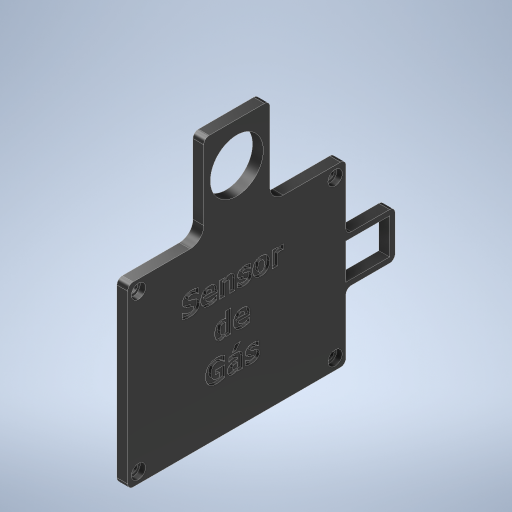
# Autodesk Inventor part: Suporte UNO-tampa
Saved by Autodesk Inventor 2023 (Build 270158000, 158)
## iProperties
Created: 2023-06-01
Part Number: Suporte UNO-tampa
Material: Genérico
Document SubType Name: Modeling
Designer: Inteli
Density: 1 g/cm^3
Appearance: Brilhosa - Preta
Author: Inteli
Autodesk Inventor part; units mm, degrees
ref_plane "YZ Plane" through (0, 0, 0) normal (1, 0, 0) x (0, 1, 0)
ref_plane "XZ Plane" through (0, 0, 0) normal (0, 1, 0) x (-1, 0, 0)
ref_plane "XY Plane" through (0, 0, 0) normal (0, 0, 1) x (1, 0, 0)
sketch "Esboço1" plane through (0, 0, 0) normal (1, 0, 0) x (0, 1, 0)
  line L0 (0, -2) -> (0, -78.8)
  line L1 (2, -80.8) -> (63.8, -80.8)
  line L2 (65.8, -78.8) -> (65.8, -52.65)
  line L3 (2, 0) -> (63.8, 0)
  line L4 (65.8, -2) -> (65.8, -28.15)
  line L5 (65.8, -28.15) -> (96.7, -28.15)
  line L6 (65.8, -52.65) -> (96.7, -52.65)
  line L7 (98.7, -50.65) -> (98.7, -30.15)
  arc A0 (98.7, -30.15) -> (96.7, -28.15) centre (96.7, -30.15) ccw
  arc A1 (96.7, -52.65) -> (98.7, -50.65) centre (96.7, -50.65) ccw
  arc A2 (65.8, -2) -> (63.8, 0) centre (63.8, -2) ccw
  arc A3 (63.8, -80.8) -> (65.8, -78.8) centre (63.8, -78.8) ccw
  arc A4 (0, -78.8) -> (2, -80.8) centre (2, -78.8) ccw
  arc A5 (2, 0) -> (0, -2) centre (2, -2) ccw
  point P0 (0, 0)
  point P1 (0, -80.8)
  point P2 (65.8, -80.8)
  point P3 (65.8, 0)
  point P4 (98.7, -28.15)
  point P5 (98.7, -52.65)
  dimension "d0" = 80.8
  dimension "d1" = 65.8
  dimension "d2" = 28.15
  dimension "d3" = 65.8
  dimension "d4" = 28.15
  dimension "d5" = 32.9
  dimension "d6" = 32.9
  dimension "d7" = 2
  constraints: 16 end point, 12 point on circle, 12 point on line, 12 tangent, 6 centre point, 5 equal radius, 4 horizontal, 2 vertical, 1 perpendicular
  measures "d0" distance of point (0, 0) point (0, -80.8)
  measures "d1" distance of point (0, -80.8) point (65.8, -80.8)
  measures "d2" distance of point (65.8, -80.8) L2.end
  measures "d3" distance of point (0, 0) point (65.8, 0)
  measures "d4" distance of point (65.8, 0) L4.end
  measures "d5" distance of L4.end point (98.7, -28.15)
  measures "d6" distance of L2.end point (98.7, -52.65)
  measures "d7" radius of A0
extrude "Extrusão1" add sketch "Esboço1" along normal blind 4
sketch "Esboço2" plane through (4, 0, 0) normal (1, 0, 0) x (0, 0, -1)
  circle A0 centre (4, 61.8) radius 1.6
  circle A1 centre (76.8, 61.8) radius 1.6
  circle A2 centre (76.8, 4) radius 1.6
  circle A3 centre (4, 4) radius 1.6
  line L0 (0, 63.8) -> (0, 2) projected
  line L1 (28.15, 65.8) -> (2, 65.8) projected
  line L2 (78.8, 65.8) -> (52.65, 65.8) projected
  line L3 (80.8, 2) -> (80.8, 63.8) projected
  line L4 (2, 0) -> (78.8, 0) projected
  circle A4 centre (40.4, 83.9) radius 9.8
  line L5 (50.65, 98.7) -> (30.15, 98.7) projected
  line L6 (52.65, 65.8) -> (52.65, 96.7) projected
  line L7 (28.15, 96.7) -> (28.15, 65.8) projected
  point P0 (0, 0)
  dimension "d10" = 3.2
  dimension "d11" = 3.2
  dimension "d12" = 3.2
  dimension "d13" = 3.2
  dimension "d14" = 4
  dimension "d15" = 4
  dimension "d16" = 4
  dimension "d17" = 4
  dimension "d18" = 4
  dimension "d19" = 4
  dimension "d20" = 4
  dimension "d21" = 4
  dimension "d22" = 19.6
  dimension "d23" = 14.8
  dimension "d24" = 24.5
  dimension "d25" = 12.25
  constraints: 5 centre point
  measures "d10" diameter of A0
  measures "d11" diameter of A1
  measures "d12" diameter of A2
  measures "d13" diameter of A3
  measures "d14" distance from line of L0 A0.centre
  measures "d15" distance from line of L1 A0.centre
  measures "d16" distance from line of L2 A1.centre
  measures "d17" distance from line of L3 A1.centre
  measures "d18" distance from line of L4 A2.centre
  measures "d19" distance from line of L3 A2.centre
  measures "d20" distance from line of L0 A3.centre
  measures "d21" distance from line of L4 A3.centre
  measures "d22" diameter of A4
  measures "d23" distance from line of L5 A4.centre
  measures "d24" distance between parallel lines of L6 L7
  measures "d25" distance from line of L6 A4.centre
extrude "Extrusão2" cut sketch "Esboço2" against normal through all
sketch "Esboço3" plane through (4, 0, 0) normal (1, 0, 0) x (0, 0, -1)
  circle A0 centre (4, 61.8) radius 1.6 projected
  circle A1 centre (4, 61.8) radius 2.6
  circle A2 centre (76.8, 61.8) radius 1.6 projected
  circle A3 centre (76.8, 61.8) radius 2.65
  circle A4 centre (76.8, 4) radius 1.6 projected
  circle A5 centre (76.8, 4) radius 2.6
  circle A6 centre (4, 4) radius 1.6 projected
  circle A7 centre (4, 4) radius 2.6
  point P0 (0, 0)
  dimension "d28" = 5.2
  dimension "d29" = 5.3
  dimension "d30" = 5.2
  dimension "d31" = 5.2
  constraints: 4 centre point, 4 coincident
  measures "d28" diameter of A1
  measures "d29" diameter of A3
  measures "d30" diameter of A5
  measures "d31" diameter of A7
extrude "Extrusão3" cut sketch "Esboço3" against normal blind 2
sketch "Esboço4" plane through (4, 0, 0) normal (1, 0, 0) x (0, 0, -1)
  line L0 (17.1867, 52.3222) -> (60.1959, 52.3222) construction
  line L1 (60.1959, 52.3222) -> (60.1959, 16.2554) construction
  line L2 (60.1959, 16.2554) -> (17.1867, 16.2554) construction
  line L3 (17.1867, 16.2554) -> (17.1867, 52.3222) construction
  spline S0 degree 2 poles (23.1095, 44.0369) (22.1889, 44.0369) (20.8015, 44.3935) (20.2051, 44.6528) knots 0 0 0 1 2 2 2
  line L4 (20.2051, 44.6528) -> (20.2051, 46.5588)
  line L5 (20.2051, 46.5588) -> (20.3866, 46.5588)
  spline S1 degree 2 poles (20.3866, 46.5588) (20.9896, 46.0467) (22.4353, 45.4956) (23.116, 45.4956) knots 0 0 0 1 2 2 2
  spline S2 degree 2 poles (23.116, 45.4956) (23.291, 45.4956) (23.855, 45.5734) (24.0236, 45.6512) knots 0 0 0 1 2 2 2
  spline S3 degree 2 poles (24.0236, 45.6512) (24.231, 45.742) (24.5228, 46.0726) (24.5228, 46.3384) knots 0 0 0 1 2 2 2
  spline S4 degree 2 poles (24.5228, 46.3384) (24.5228, 46.6431) (24.0495, 47.0191) (23.7254, 47.1034) knots 0 0 0 1 2 2 2
  spline S5 degree 2 poles (23.7254, 47.1034) (23.3169, 47.2136) (22.3899, 47.4016) (21.9814, 47.5442) knots 0 0 0 1 2 2 2
  spline S6 degree 2 poles (21.9814, 47.5442) (21.0544, 47.8684) (20.2505, 48.977) (20.2505, 49.8068) knots 0 0 0 1 2 2 2
  spline S7 degree 2 poles (20.2505, 49.8068) (20.2505, 50.9284) (22.15, 52.3222) (23.5763, 52.3222) knots 0 0 0 1 2 2 2
  spline S8 degree 2 poles (23.5763, 52.3222) (24.2894, 52.3222) (25.7027, 52.0305) (26.2602, 51.7841) knots 0 0 0 1 2 2 2
  line L6 (26.2602, 51.7841) -> (26.2602, 49.9559)
  line L7 (26.2602, 49.9559) -> (26.0852, 49.9559)
  spline S9 degree 2 poles (26.0852, 49.9559) (25.6379, 50.3384) (24.3542, 50.8635) (23.68, 50.8635) knots 0 0 0 1 2 2 2
  spline S10 degree 2 poles (23.68, 50.8635) (23.4142, 50.8635) (22.9993, 50.7857) (22.7659, 50.682) knots 0 0 0 1 2 2 2
  spline S11 degree 2 poles (22.7659, 50.682) (22.5779, 50.5977) (22.3056, 50.2606) (22.3056, 50.0532) knots 0 0 0 1 2 2 2
  spline S12 degree 2 poles (22.3056, 50.0532) (22.3056, 49.742) (22.74, 49.3854) (23.3623, 49.2428) knots 0 0 0 1 2 2 2
  spline S13 degree 2 poles (23.3623, 49.2428) (23.7643, 49.152) (24.5098, 48.977) (24.9377, 48.8279) knots 0 0 0 1 2 2 2
  spline S14 degree 2 poles (24.9377, 48.8279) (25.7675, 48.5232) (26.5779, 47.5118) (26.5779, 46.682) knots 0 0 0 1 2 2 2
  spline S15 degree 2 poles (26.5779, 46.682) (26.5779, 45.4891) (24.7043, 44.0369) (23.1095, 44.0369) knots 0 0 0 1 2 2 2
  spline S16 degree 2 poles (30.5908, 44.0175) (28.8793, 44.0175) (27.0576, 45.6512) (27.0576, 47.1617) knots 0 0 0 1 2 2 2
  spline S17 degree 2 poles (27.0576, 47.1617) (27.0576, 48.6399) (28.7562, 50.4032) (30.2861, 50.4032) knots 0 0 0 1 2 2 2
  spline S18 degree 2 poles (30.2861, 50.4032) (31.667, 50.4032) (33.0673, 48.9057) (33.0673, 47.5183) knots 0 0 0 1 2 2 2
  line L8 (33.0673, 47.5183) -> (33.0673, 46.8376)
  line L9 (33.0673, 46.8376) -> (28.9377, 46.8376)
  spline S19 degree 2 poles (28.9377, 46.8376) (28.9636, 46.4162) (29.2683, 45.8587) (29.5147, 45.6901) knots 0 0 0 1 2 2 2
  spline S20 degree 2 poles (29.5147, 45.6901) (29.7545, 45.5216) (30.4028, 45.3789) (30.7853, 45.3789) knots 0 0 0 1 2 2 2
  spline S21 degree 2 poles (30.7853, 45.3789) (31.1095, 45.3789) (31.7448, 45.5216) (32.0106, 45.6447) knots 0 0 0 1 2 2 2
  spline S22 degree 2 poles (32.0106, 45.6447) (32.244, 45.742) (32.633, 45.9818) (32.7562, 46.0726) knots 0 0 0 1 2 2 2
  line L10 (32.7562, 46.0726) -> (32.9571, 46.0726)
  line L11 (32.9571, 46.0726) -> (32.9571, 44.5167)
  spline S23 degree 2 poles (32.9571, 44.5167) (32.7238, 44.4259) (32.3477, 44.2703) (32.0106, 44.1925) knots 0 0 0 1 2 2 2
  spline S24 degree 2 poles (32.0106, 44.1925) (31.7059, 44.1083) (31.0576, 44.0175) (30.5908, 44.0175) knots 0 0 0 1 2 2 2
  spline S25 degree 2 poles (31.2132, 47.9721) (31.2003, 48.5686) (30.6751, 49.1974) (30.137, 49.1974) knots 0 0 0 1 2 2 2
  spline S26 degree 2 poles (30.137, 49.1974) (29.586, 49.1974) (28.9636, 48.5361) (28.9312, 47.9721) knots 0 0 0 1 2 2 2
  line L12 (28.9312, 47.9721) -> (31.2132, 47.9721)
  line L13 (39.68, 44.1796) -> (37.787, 44.1796)
  line L14 (37.787, 44.1796) -> (37.787, 47.1682)
  spline S27 degree 2 poles (37.787, 47.1682) (37.787, 47.5378) (37.7286, 48.2639) (37.6508, 48.4324) knots 0 0 0 1 2 2 2
  spline S28 degree 2 poles (37.6508, 48.4324) (37.5536, 48.6399) (37.1905, 48.8149) (36.8793, 48.8149) knots 0 0 0 1 2 2 2
  spline S29 degree 2 poles (36.8793, 48.8149) (36.6524, 48.8149) (36.1792, 48.6399) (35.9134, 48.4519) knots 0 0 0 1 2 2 2
  line L15 (35.9134, 48.4519) -> (35.9134, 44.1796)
  line L16 (35.9134, 44.1796) -> (34.0333, 44.1796)
  line L17 (34.0333, 44.1796) -> (34.0333, 50.2152)
  line L18 (34.0333, 50.2152) -> (35.9134, 50.2152)
  line L19 (35.9134, 50.2152) -> (35.9134, 49.5475)
  spline S30 degree 2 poles (35.9134, 49.5475) (36.3737, 49.9365) (37.2489, 50.3773) (37.7805, 50.3773) knots 0 0 0 1 2 2 2
  spline S31 degree 2 poles (37.7805, 50.3773) (38.7011, 50.3773) (39.68, 49.2104) (39.68, 48.1083) knots 0 0 0 1 2 2 2
  line L20 (39.68, 48.1083) -> (39.68, 44.1796)
  spline S32 degree 2 poles (42.9085, 44.0175) (42.2473, 44.0175) (41.0609, 44.3092) (40.6719, 44.5037) knots 0 0 0 1 2 2 2
  line L21 (40.6719, 44.5037) -> (40.6719, 46.0921)
  line L22 (40.6719, 46.0921) -> (40.8275, 46.0921)
  spline S33 degree 2 poles (40.8275, 46.0921) (40.9636, 45.9883) (41.3072, 45.742) (41.6119, 45.6058) knots 0 0 0 1 2 2 2
  spline S34 degree 2 poles (41.6119, 45.6058) (41.8777, 45.4827) (42.5325, 45.3076) (42.9215, 45.3076) knots 0 0 0 1 2 2 2
  spline S35 degree 2 poles (42.9215, 45.3076) (43.3169, 45.3076) (43.9263, 45.554) (43.9263, 45.8198) knots 0 0 0 1 2 2 2
  spline S36 degree 2 poles (43.9263, 45.8198) (43.9263, 46.0272) (43.6476, 46.2476) (43.2456, 46.3384) knots 0 0 0 1 2 2 2
  spline S37 degree 2 poles (43.2456, 46.3384) (43.0317, 46.3968) (42.3769, 46.5199) (42.1241, 46.5977) knots 0 0 0 1 2 2 2
  spline S38 degree 2 poles (42.1241, 46.5977) (41.4109, 46.8181) (40.6978, 47.6804) (40.6978, 48.387) knots 0 0 0 1 2 2 2
  spline S39 degree 2 poles (40.6978, 48.387) (40.6978, 48.789) (41.0673, 49.5021) (41.4304, 49.7809) knots 0 0 0 1 2 2 2
  spline S40 degree 2 poles (41.4304, 49.7809) (41.787, 50.0532) (42.8437, 50.3773) (43.5114, 50.3773) knots 0 0 0 1 2 2 2
  spline S41 degree 2 poles (43.5114, 50.3773) (44.1468, 50.3773) (45.21, 50.1245) (45.573, 49.9494) knots 0 0 0 1 2 2 2
  line L23 (45.573, 49.9494) -> (45.573, 48.4194)
  line L24 (45.573, 48.4194) -> (45.4239, 48.4194)
  spline S42 degree 2 poles (45.4239, 48.4194) (45.3267, 48.4972) (44.9053, 48.7501) (44.7108, 48.8408) knots 0 0 0 1 2 2 2
  spline S43 degree 2 poles (44.7108, 48.8408) (44.4709, 48.9446) (43.8874, 49.0872) (43.5827, 49.0872) knots 0 0 0 1 2 2 2
  spline S44 degree 2 poles (43.5827, 49.0872) (43.1743, 49.0872) (42.6103, 48.8084) (42.6103, 48.5815) knots 0 0 0 1 2 2 2
  spline S45 degree 2 poles (42.6103, 48.5815) (42.6103, 48.3741) (42.8891, 48.1407) (43.3558, 48.024) knots 0 0 0 1 2 2 2
  spline S46 degree 2 poles (43.3558, 48.024) (43.5957, 47.9656) (44.2246, 47.8554) (44.5163, 47.7582) knots 0 0 0 1 2 2 2
  spline S47 degree 2 poles (44.5163, 47.7582) (45.1646, 47.5507) (45.8388, 46.7404) (45.8388, 46.0661) knots 0 0 0 1 2 2 2
  spline S48 degree 2 poles (45.8388, 46.0661) (45.8388, 45.6447) (45.4434, 44.8733) (45.0738, 44.6139) knots 0 0 0 1 2 2 2
  spline S49 degree 2 poles (45.0738, 44.6139) (44.6913, 44.3287) (43.6411, 44.0175) (42.9085, 44.0175) knots 0 0 0 1 2 2 2
  spline S50 degree 2 poles (52.5228, 47.1942) (52.5228, 45.7031) (50.8956, 43.9916) (49.4109, 43.9916) knots 0 0 0 1 2 2 2
  spline S51 degree 2 poles (49.4109, 43.9916) (47.9328, 43.9916) (46.2926, 45.7031) (46.2926, 47.1942) knots 0 0 0 1 2 2 2
  spline S52 degree 2 poles (46.2926, 47.1942) (46.2926, 48.6982) (47.9328, 50.4032) (49.4109, 50.4032) knots 0 0 0 1 2 2 2
  spline S53 degree 2 poles (49.4109, 50.4032) (50.8891, 50.4032) (52.5228, 48.6917) (52.5228, 47.1942) knots 0 0 0 1 2 2 2
  spline S54 degree 2 poles (50.5973, 47.1812) (50.5973, 47.7193) (50.4223, 48.4389) (50.2667, 48.6528) knots 0 0 0 1 2 2 2
  spline S55 degree 2 poles (50.2667, 48.6528) (50.0981, 48.8797) (49.6767, 49.0548) (49.4109, 49.0548) knots 0 0 0 1 2 2 2
  spline S56 degree 2 poles (49.4109, 49.0548) (49.1516, 49.0548) (48.7432, 48.8992) (48.5746, 48.6788) knots 0 0 0 1 2 2 2
  spline S57 degree 2 poles (48.5746, 48.6788) (48.4126, 48.4713) (48.2181, 47.7387) (48.2181, 47.1812) knots 0 0 0 1 2 2 2
  spline S58 degree 2 poles (48.2181, 47.1812) (48.2181, 46.6301) (48.3996, 45.9494) (48.5487, 45.742) knots 0 0 0 1 2 2 2
  spline S59 degree 2 poles (48.5487, 45.742) (48.6978, 45.5345) (49.1516, 45.34) (49.4239, 45.34) knots 0 0 0 1 2 2 2
  spline S60 degree 2 poles (49.4239, 45.34) (49.6508, 45.34) (50.1176, 45.5345) (50.2602, 45.729) knots 0 0 0 1 2 2 2
  spline S61 degree 2 poles (50.2602, 45.729) (50.4223, 45.9559) (50.5973, 46.6107) (50.5973, 47.1812) knots 0 0 0 1 2 2 2
  line L25 (57.573, 48.4324) -> (57.4174, 48.4324)
  spline S62 degree 2 poles (57.4174, 48.4324) (57.3072, 48.4713) (56.8988, 48.5102) (56.6524, 48.5102) knots 0 0 0 1 2 2 2
  spline S63 degree 2 poles (56.6524, 48.5102) (56.3607, 48.5102) (55.7059, 48.3352) (55.4012, 48.2185) knots 0 0 0 1 2 2 2
  line L26 (55.4012, 48.2185) -> (55.4012, 44.1796)
  line L27 (55.4012, 44.1796) -> (53.5212, 44.1796)
  line L28 (53.5212, 44.1796) -> (53.5212, 50.2152)
  line L29 (53.5212, 50.2152) -> (55.4012, 50.2152)
  line L30 (55.4012, 50.2152) -> (55.4012, 49.3465)
  spline S64 degree 2 poles (55.4012, 49.3465) (55.5309, 49.4632) (55.9847, 49.8263) (56.1727, 49.9365) knots 0 0 0 1 2 2 2
  spline S65 degree 2 poles (56.1727, 49.9365) (56.3802, 50.0596) (56.9247, 50.2347) (57.1646, 50.2347) knots 0 0 0 1 2 2 2
  spline S66 degree 2 poles (57.1646, 50.2347) (57.2554, 50.2347) (57.4823, 50.2217) (57.573, 50.2152) knots 0 0 0 1 2 2 2
  line L31 (57.573, 50.2152) -> (57.573, 48.4324)
  line L32 (38.1662, 31.0078) -> (36.2861, 31.0078)
  line L33 (36.2861, 31.0078) -> (36.2861, 31.6366)
  spline S67 degree 2 poles (36.2861, 31.6366) (36.1046, 31.4875) (35.6379, 31.1439) (35.4563, 31.0532) knots 0 0 0 1 2 2 2
  spline S68 degree 2 poles (35.4563, 31.0532) (35.2359, 30.9494) (34.7951, 30.8392) (34.4904, 30.8392) knots 0 0 0 1 2 2 2
  spline S69 degree 2 poles (34.4904, 30.8392) (33.4596, 30.8392) (32.2537, 32.5507) (32.2537, 33.977) knots 0 0 0 1 2 2 2
  spline S70 degree 2 poles (32.2537, 33.977) (32.2537, 34.7679) (32.6622, 35.9284) (33.0187, 36.3562) knots 0 0 0 1 2 2 2
  spline S71 degree 2 poles (33.0187, 36.3562) (33.3494, 36.7517) (34.2829, 37.2055) (34.8015, 37.2055) knots 0 0 0 1 2 2 2
  spline S72 degree 2 poles (34.8015, 37.2055) (35.2748, 37.2055) (35.8842, 37.0045) (36.2861, 36.7971) knots 0 0 0 1 2 2 2
  line L34 (36.2861, 36.7971) -> (36.2861, 39.3643)
  line L35 (36.2861, 39.3643) -> (38.1662, 39.3643)
  line L36 (38.1662, 39.3643) -> (38.1662, 31.0078)
  line L37 (36.2861, 32.6674) -> (36.2861, 35.6302)
  spline S73 degree 2 poles (36.2861, 35.6302) (36.15, 35.7015) (35.6962, 35.7922) (35.5341, 35.7922) knots 0 0 0 1 2 2 2
  spline S74 degree 2 poles (35.5341, 35.7922) (34.8599, 35.7922) (34.1792, 34.8457) (34.1792, 33.9964) knots 0 0 0 1 2 2 2
  spline S75 degree 2 poles (34.1792, 33.9964) (34.1792, 33.1018) (34.7238, 32.3044) (35.3267, 32.3044) knots 0 0 0 1 2 2 2
  spline S76 degree 2 poles (35.3267, 32.3044) (35.573, 32.3044) (36.0787, 32.4989) (36.2861, 32.6674) knots 0 0 0 1 2 2 2
  spline S77 degree 2 poles (42.6978, 30.8457) (40.9863, 30.8457) (39.1646, 32.4794) (39.1646, 33.99) knots 0 0 0 1 2 2 2
  spline S78 degree 2 poles (39.1646, 33.99) (39.1646, 35.4681) (40.8631, 37.2314) (42.3931, 37.2314) knots 0 0 0 1 2 2 2
  spline S79 degree 2 poles (42.3931, 37.2314) (43.774, 37.2314) (45.1743, 35.7339) (45.1743, 34.3465) knots 0 0 0 1 2 2 2
  line L38 (45.1743, 34.3465) -> (45.1743, 33.6658)
  line L39 (45.1743, 33.6658) -> (41.0447, 33.6658)
  spline S80 degree 2 poles (41.0447, 33.6658) (41.0706, 33.2444) (41.3753, 32.6869) (41.6216, 32.5183) knots 0 0 0 1 2 2 2
  spline S81 degree 2 poles (41.6216, 32.5183) (41.8615, 32.3498) (42.5098, 32.2071) (42.8923, 32.2071) knots 0 0 0 1 2 2 2
  spline S82 degree 2 poles (42.8923, 32.2071) (43.2165, 32.2071) (43.8518, 32.3498) (44.1176, 32.4729) knots 0 0 0 1 2 2 2
  spline S83 degree 2 poles (44.1176, 32.4729) (44.351, 32.5702) (44.74, 32.8101) (44.8631, 32.9008) knots 0 0 0 1 2 2 2
  line L40 (44.8631, 32.9008) -> (45.0641, 32.9008)
  line L41 (45.0641, 32.9008) -> (45.0641, 31.3449)
  spline S84 degree 2 poles (45.0641, 31.3449) (44.8307, 31.2541) (44.4547, 31.0985) (44.1176, 31.0208) knots 0 0 0 1 2 2 2
  spline S85 degree 2 poles (44.1176, 31.0208) (43.8129, 30.9365) (43.1646, 30.8457) (42.6978, 30.8457) knots 0 0 0 1 2 2 2
  spline S86 degree 2 poles (43.3202, 34.8003) (43.3072, 35.3968) (42.7821, 36.0256) (42.244, 36.0256) knots 0 0 0 1 2 2 2
  spline S87 degree 2 poles (42.244, 36.0256) (41.693, 36.0256) (41.0706, 35.3643) (41.0382, 34.8003) knots 0 0 0 1 2 2 2
  line L42 (41.0382, 34.8003) -> (43.3202, 34.8003)
  spline S88 degree 2 poles (35.9782, 18.2898) (35.4531, 18.0759) (33.774, 17.6674) (32.9571, 17.6674) knots 0 0 0 1 2 2 2
  spline S89 degree 2 poles (32.9571, 17.6674) (31.0706, 17.6674) (28.834, 19.8457) (28.834, 21.8425) knots 0 0 0 1 2 2 2
  spline S90 degree 2 poles (28.834, 21.8425) (28.834, 23.7225) (31.0706, 25.9916) (33.0155, 25.9916) knots 0 0 0 1 2 2 2
  spline S91 degree 2 poles (33.0155, 25.9916) (34.0203, 25.9916) (35.278, 25.6091) (35.9458, 25.2849) knots 0 0 0 1 2 2 2
  line L43 (35.9458, 25.2849) -> (35.9458, 23.4049)
  line L44 (35.9458, 23.4049) -> (35.7643, 23.4049)
  spline S92 degree 2 poles (35.7643, 23.4049) (35.6216, 23.5151) (35.0771, 23.9365) (34.8178, 24.0791) knots 0 0 0 1 2 2 2
  spline S93 degree 2 poles (34.8178, 24.0791) (34.5195, 24.2541) (33.7286, 24.5005) (33.2878, 24.5005) knots 0 0 0 1 2 2 2
  spline S94 degree 2 poles (33.2878, 24.5005) (32.7756, 24.5005) (31.9263, 24.1764) (31.5957, 23.8457) knots 0 0 0 1 2 2 2
  spline S95 degree 2 poles (31.5957, 23.8457) (31.278, 23.5216) (30.9085, 22.5297) (30.9085, 21.8749) knots 0 0 0 1 2 2 2
  spline S96 degree 2 poles (30.9085, 21.8749) (30.9085, 20.4746) (32.3153, 19.1391) (33.5276, 19.1391) knots 0 0 0 1 2 2 2
  spline S97 degree 2 poles (33.5276, 19.1391) (33.6379, 19.1391) (33.9231, 19.152) (34.0333, 19.1585) knots 0 0 0 1 2 2 2
  line L45 (34.0333, 19.1585) -> (34.0333, 20.7339)
  line L46 (34.0333, 20.7339) -> (32.4839, 20.7339)
  line L47 (32.4839, 20.7339) -> (32.4839, 22.2315)
  line L48 (32.4839, 22.2315) -> (35.9782, 22.2315)
  line L49 (35.9782, 22.2315) -> (35.9782, 18.2898)
  spline S98 degree 2 poles (40.7108, 18.4778) (40.5163, 18.3157) (40.2116, 18.0564) (39.9523, 17.9268) knots 0 0 0 1 2 2 2
  spline S99 degree 2 poles (39.9523, 17.9268) (39.6994, 17.8036) (39.2197, 17.6739) (38.7918, 17.6739) knots 0 0 0 1 2 2 2
  spline S100 degree 2 poles (38.7918, 17.6739) (37.9879, 17.6739) (36.9312, 18.7501) (36.9312, 19.567) knots 0 0 0 1 2 2 2
  spline S101 degree 2 poles (36.9312, 19.567) (36.9312, 20.2347) (37.4693, 21.0645) (37.975, 21.3044) knots 0 0 0 1 2 2 2
  spline S102 degree 2 poles (37.975, 21.3044) (38.4871, 21.5507) (39.9069, 21.7452) (40.7238, 21.7971) knots 0 0 0 1 2 2 2
  line L50 (40.7238, 21.7971) -> (40.7238, 21.8295)
  spline S103 degree 2 poles (40.7238, 21.8295) (40.7238, 22.3287) (39.9847, 22.7112) (39.2456, 22.7112) knots 0 0 0 1 2 2 2
  spline S104 degree 2 poles (39.2456, 22.7112) (38.915, 22.7112) (38.0203, 22.4713) (37.599, 22.2833) knots 0 0 0 1 2 2 2
  line L51 (37.599, 22.2833) -> (37.4369, 22.2833)
  line L52 (37.4369, 22.2833) -> (37.4369, 23.742)
  spline S105 degree 2 poles (37.4369, 23.742) (37.7156, 23.8198) (38.9604, 24.0402) (39.5957, 24.0402) knots 0 0 0 1 2 2 2
  spline S106 degree 2 poles (39.5957, 24.0402) (41.1516, 24.0402) (42.5779, 23.0029) (42.5779, 21.9397) knots 0 0 0 1 2 2 2
  line L53 (42.5779, 21.9397) -> (42.5779, 17.836)
  line L54 (42.5779, 17.836) -> (40.7108, 17.836)
  line L55 (40.7108, 17.836) -> (40.7108, 18.4778)
  line L56 (41.6184, 26.8409) -> (40.0041, 24.7274)
  line L57 (40.0041, 24.7274) -> (38.727, 24.7274)
  line L58 (38.727, 24.7274) -> (39.8421, 26.8409)
  line L59 (39.8421, 26.8409) -> (41.6184, 26.8409)
  line L60 (40.7108, 19.4114) -> (40.7108, 20.6626)
  spline S107 degree 2 poles (40.7108, 20.6626) (40.231, 20.6172) (39.6411, 20.5459) (39.3558, 20.4422) knots 0 0 0 1 2 2 2
  spline S108 degree 2 poles (39.3558, 20.4422) (39.103, 20.3579) (38.8307, 20.0078) (38.8307, 19.7225) knots 0 0 0 1 2 2 2
  spline S109 degree 2 poles (38.8307, 19.7225) (38.8307, 19.3012) (39.291, 18.9835) (39.7383, 18.9835) knots 0 0 0 1 2 2 2
  spline S110 degree 2 poles (39.7383, 18.9835) (39.9847, 18.9835) (40.5033, 19.2104) (40.7108, 19.4114) knots 0 0 0 1 2 2 2
  spline S111 degree 2 poles (45.8064, 17.6739) (45.1451, 17.6739) (43.9588, 17.9657) (43.5698, 18.1601) knots 0 0 0 1 2 2 2
  line L61 (43.5698, 18.1601) -> (43.5698, 19.7485)
  line L62 (43.5698, 19.7485) -> (43.7254, 19.7485)
  spline S112 degree 2 poles (43.7254, 19.7485) (43.8615, 19.6447) (44.2051, 19.3984) (44.5098, 19.2623) knots 0 0 0 1 2 2 2
  spline S113 degree 2 poles (44.5098, 19.2623) (44.7756, 19.1391) (45.4304, 18.964) (45.8194, 18.964) knots 0 0 0 1 2 2 2
  spline S114 degree 2 poles (45.8194, 18.964) (46.2148, 18.964) (46.8242, 19.2104) (46.8242, 19.4762) knots 0 0 0 1 2 2 2
  spline S115 degree 2 poles (46.8242, 19.4762) (46.8242, 19.6836) (46.5455, 19.9041) (46.1435, 19.9948) knots 0 0 0 1 2 2 2
  spline S116 degree 2 poles (46.1435, 19.9948) (45.9296, 20.0532) (45.2748, 20.1764) (45.022, 20.2541) knots 0 0 0 1 2 2 2
  spline S117 degree 2 poles (45.022, 20.2541) (44.3088, 20.4746) (43.5957, 21.3368) (43.5957, 22.0435) knots 0 0 0 1 2 2 2
  spline S118 degree 2 poles (43.5957, 22.0435) (43.5957, 22.4454) (43.9652, 23.1585) (44.3283, 23.4373) knots 0 0 0 1 2 2 2
  spline S119 degree 2 poles (44.3283, 23.4373) (44.6849, 23.7096) (45.7416, 24.0337) (46.4093, 24.0337) knots 0 0 0 1 2 2 2
  spline S120 degree 2 poles (46.4093, 24.0337) (47.0447, 24.0337) (48.1079, 23.7809) (48.4709, 23.6059) knots 0 0 0 1 2 2 2
  line L63 (48.4709, 23.6059) -> (48.4709, 22.0759)
  line L64 (48.4709, 22.0759) -> (48.3218, 22.0759)
  spline S121 degree 2 poles (48.3218, 22.0759) (48.2246, 22.1537) (47.8032, 22.4065) (47.6087, 22.4973) knots 0 0 0 1 2 2 2
  spline S122 degree 2 poles (47.6087, 22.4973) (47.3688, 22.601) (46.7853, 22.7436) (46.4806, 22.7436) knots 0 0 0 1 2 2 2
  spline S123 degree 2 poles (46.4806, 22.7436) (46.0722, 22.7436) (45.5082, 22.4648) (45.5082, 22.2379) knots 0 0 0 1 2 2 2
  spline S124 degree 2 poles (45.5082, 22.2379) (45.5082, 22.0305) (45.787, 21.7971) (46.2537, 21.6804) knots 0 0 0 1 2 2 2
  spline S125 degree 2 poles (46.2537, 21.6804) (46.4936, 21.6221) (47.1225, 21.5118) (47.4142, 21.4146) knots 0 0 0 1 2 2 2
  spline S126 degree 2 poles (47.4142, 21.4146) (48.0625, 21.2071) (48.7367, 20.3968) (48.7367, 19.7225) knots 0 0 0 1 2 2 2
  spline S127 degree 2 poles (48.7367, 19.7225) (48.7367, 19.3012) (48.3413, 18.5297) (47.9717, 18.2704) knots 0 0 0 1 2 2 2
  spline S128 degree 2 poles (47.9717, 18.2704) (47.5892, 17.9851) (46.539, 17.6739) (45.8064, 17.6739) knots 0 0 0 1 2 2 2
  point P0 (0, 0)
  constraints: 2 other
extrude "Extrusão4" cut sketch "Esboço4" against normal blind 1
fillet "Arredondamento1" radius 5 2 edges at (2, 65.8, -52.65) (2, 65.8, -28.15)
sketch "Esboço5" plane through (4, 0, 0) normal (1, 0, 0) x (0, 0, -1)
  line L0 (80.8, 2) -> (80.8, 63.8) projected
  line L1 (80.8, 41.5) -> (99, 41.5)
  line L2 (99, 41.5) -> (99, 24.3)
  line L3 (99, 24.3) -> (80.8, 24.3)
  line L4 (80.8, 24.3) -> (80.8, 41.5)
  line L5 (2, 0) -> (78.8, 0) projected
  line L6 (78.8, 65.8) -> (57.65, 65.8) projected
  point P0 (0, 0)
  point P1 (68.225, 65.8)
  dimension "d37" = 18.2
  dimension "d38" = 17.2
  dimension "d39" = 65.8
  dimension "d40" = 24.3
  constraints: 8 end point, 2 parallel, 1 horizontal, 1 midpoint, 1 perpendicular, 1 point on line
  measures "d37" distance of L2.end L3.end
  measures "d38" distance of L1.end L2.end
  measures "d39" distance between parallel lines of L5 L6
  measures "d40" distance from line of L1 point (68.225, 65.8)
extrude "Extrusão5" add sketch "Esboço5" against normal blind 4
fillet "Arredondamento2" radius 2 4 edges at (2, 41.5, -80.8) (2, 24.3, -80.8) (2, 41.5, -99) (2, 24.3, -99)
sketch "Esboço6" plane through (4, 0, 0) normal (1, 0, 0) x (0, 0, -1)
  line L0 (80.8, 39.5) -> (97, 39.5)
  line L1 (97, 39.5) -> (97, 26.3)
  line L2 (97, 26.3) -> (80.8, 26.3)
  line L3 (80.8, 26.3) -> (80.8, 39.5)
  line L4 (97, 41.5) -> (82.8, 41.5) projected
  line L5 (99, 26.3) -> (99, 39.5) projected
  point P0 (0, 0)
  dimension "d44" = 16.2
  dimension "d45" = 13.2
  dimension "d46" = 2
  dimension "d47" = 2
  constraints: 8 end point, 2 parallel, 1 horizontal, 1 perpendicular
  measures "d44" distance of L1.end L2.end
  measures "d45" distance of L0.end L1.end
  measures "d46" distance between parallel lines of L4 L0
  measures "d47" distance between parallel lines of L5 L1
extrude "Extrusão6" cut sketch "Esboço6" against normal blind 4
equation "\"d25\" = 0.5 * d24"
equation "\"d40\" = -0.5 * d38 + 0.5 * d39"
